Autodesk Fusion 360 part; units mm, degrees
(part 6 of 6)
  arc A719 (142.7278, 4.1602) -> (143.1708, 4.6744) centre (142.6711, 4.657) ccw
  circle A720 centre (0, 0) radius 145
  dimension "d16" = 290
  constraint coincident A720.centre origin
  measures "d16" diameter of A720
extrude "Extrude3" add sketch "Sketch3" along normal blind 2 contours L0 A0 A1 A2 A3 L1 A4 A5 A6 A7 L2 A8 A9 A10 A11 L3 A12 A13 A14 A15 L4 A16 A17 A18 A19 L5 A20 A21 A22 A23 L6 A24 A25 A26 A27 L7 A28 A29 A30 A31 L8 A32 A33 A34 A35 L9 A36 A37 A38 A39 L10 A40 A41 A42 A43 L11 A44 A45 A46 A47 L12 A48 A49 A50 A51 L13 A52 A53 A54 A55 L14 A56 A57 A58 A59 L15 A60 A61 A62 A63 L16 A64 A65 A66 A67 L17 A68 A69 A70 A71 L18 A72 A73 A74 A75 L19 A76 A77 A78 A79 L20 A80 A81 A82 A83 L21 A84 A85 A86 A87 L22 A88 A89 A90 A91 L23 A92 A93 A94 A95 L24 A96 A97 A98 A99 L25 A100 A101 A102 A103 L26 A104 A105 A106 A107 L27 A108 A109 A110 A111 L28 A112 A113 A114 A115 L29 A116 A117 A118 A119 L30 A120 A121 A122 A123 L31 A124 A125 A126 A127 L32 A128 A129 A130 A131 L33 A132 A133 A134 A135 L34 A136 A137 A138 A139 L35 A140 A141 A142 A143 L36 A144 A145 A146 A147 L37 A148 A149 A150 A151 L38 A152 A153 A154 A155 L39 A156 A157 A158 A159 L40 A160 A161 A162 A163 L41 A164 A165 A166 A167 L42 A168 A169 A170 A171 L43 A172 A173 A174 A175 L44 A176 A177 A178 A179 L45 A180 A181 A182 A183 L46 A184 A185 A186 A187 L47 A188 A189 A190 A191 L48 A192 A193 A194 A195 L49 A196 A197 A198 A199 L50 A200 A201 A202 A203 L51 A204 A205 A206 A207 L52 A208 A209 A210 A211 L53 A212 A213 A214 A215 L54 A216 A217 A218 A219 L55 A220 A221 A222 A223 L56 A224 A225 A226 A227 L57 A228 A229 A230 A231 L58 A232 A233 A234 A235 L59 A236 A237 A238 A239 L60 A240 A241 A242 A243 L61 A244 A245 A246 A247 L62 A248 A249 A250 A251 L63 A252 A253 A254 A255 L64 A256 A257 A258 A259 L65 A260 A261 A262 A263 L66 A264 A265 A266 A267 L67 A268 A269 A270 A271 L68 A272 A273 A274 A275 L69 A276 A277 A278 A279 L70 A280 A281 A282 A283 L71 A284 A285 A286 A287 L72 A288 A289 A290 A291 L73 A292 A293 A294 A295 L74 A296 A297 A298 A299 L75 A300 A301 A302 A303 L76 A304 A305 A306 A307 L77 A308 A309 A310 A311 L78 A312 A313 A314 A315 L79 A316 A317 A318 A319 L80 A320 A321 A322 A323 L81 A324 A325 A326 A327 L82 A328 A329 A330 A331 L83 A332 A333 A334 A335 L84 A336 A337 A338 A339 L85 A340 A341 A342 A343 L86 A344 A345 A346 A347 L87 A348 A349 A350 A351 L88 A352 A353 A354 A355 L89 A356 A357 A358 A359 L90 A360 A361 A362 A363 L91 A364 A365 A366 A367 L92 A368 A369 A370 A371 L93 A372 A373 A374 A375 L94 A376 A377 A378 A379 L95 A380 A381 A382 A383 L96 A384 A385 A386 A387 L97 A388 A389 A390 A391 L98 A392 A393 A394 A395 L99 A396 A397 A398 A399 L100 A400 A401 A402 A403 L101 A404 A405 A406 A407 L102 A408 A409 A410 A411 L103 A412 A413 A414 A415 L104 A416 A417 A418 A419 L105 A420 A421 A422 A423 L106 A424 A425 A426 A427 L107 A428 A429 A430 A431 L108 A432 A433 A434 A435 L109 A436 A437 A438 A439 L110 A440 A441 A442 A443 L111 A444 A445 A446 A447 L112 A448 A449 A450 A451 L113 A452 A453 A454 A455 L114 A456 A457 A458 A459 L115 A460 A461 A462 A463 L116 A464 A465 A466 A467 L117 A468 A469 A470 A471 L118 A472 A473 A474 A475 L119 A476 A477 A478 A479 L120 A480 A481 A482 A483 L121 A484 A485 A486 A487 L122 A488 A489 A490 A491 L123 A492 A493 A494 A495 L124 A496 A497 A498 A499 L125 A500 A501 A502 A503 L126 A504 A505 A506 A507 L127 A508 A509 A510 A511 L128 A512 A513 A514 A515 L129 A516 A517 A518 A519 L130 A520 A521 A522 A523 L131 A524 A525 A526 A527 L132 A528 A529 A530 A531 L133 A532 A533 A534 A535 L134 A536 A537 A538 A539 L135 A540 A541 A542 A543 L136 A544 A545 A546 A547 L137 A548 A549 A550 A551 L138 A552 A553 A554 A555 L139 A556 A557 A558 A559 L140 A560 A561 A562 A563 L141 A564 A565 A566 A567 L142 A568 A569 A570 A571 L143 A572 A573 A574 A575 L144 A576 A577 A578 A579 L145 A580 A581 A582 A583 L146 A584 A585 A586 A587 L147 A588 A589 A590 A591 L148 A592 A593 A594 A595 L149 A596 A597 A598 A599 L150 A600 A601 A602 A603 L151 A604 A605 A606 A607 L152 A608 A609 A610 A611 L153 A612 A613 A614 A615 L154 A616 A617 A618 A619 L155 A620 A621 A622 A623 L156 A624 A625 A626 A627 L157 A628 A629 A630 A631 L158 A632 A633 A634 A635 L159 A636 A637 A638 A639 L160 A640 A641 A642 A643 L161 A644 A645 A646 A647 L162 A648 A649 A650 A651 L163 A652 A653 A654 A655 L164 A656 A657 A658 A659 L165 A660 A661 A662 A663 L166 A664 A665 A666 A667 L167 A668 A669 A670 A671 L168 A672 A673 A674 A675 L169 A676 A677 A678 A679 L170 A680 A681 A682 A683 L171 A684 A685 A686 A687 L172 A688 A689 A690 A691 L173 A692 A693 A694 A695 L174 A696 A697 A698 A699 L175 A700 A701 A702 A703 L176 A704 A705 A706 A707 L177 A708 A709 A710 A711 L178 A712 A713 A714 A715 L179 A716 A717 A718 A719 | A720
chamfer "Chamfer1" distance 1.5 angle 45 2 edges at (135.1875, 52.4342, 16) (-135.1875, 52.4342, 0)
sketch "Sketch4" plane through (0, 0, 18) normal (0, 0, 1) x (-1, 0, 0)
  circle A0 centre (0, 0) radius 145
  circle A1 centre (0, 0) radius 110
  dimension "d19" = 220
  constraint coincident A0.centre A1.centre
  measures "d19" diameter of A1
extrude "Extrude4" cut sketch "Sketch4" against normal blind 40 contours A1
sketch "Sketch5" plane through (0, 0, 18) normal (0, 0, 1) x (-1, 0, 0)
  circle A0 centre (0, 0) radius 110
  circle A1 centre (0, 0) radius 145
  line L0 (0, 0) -> (0, -252.5866) construction
  line L1 (0, 0) -> (0, -4.3982) construction
  line L2 (0, 0) -> (-17.5, -126.2933) construction
  line L3 (0, 0) -> (17.5, -126.2933) construction
  circle A2 centre (0, 0) radius 127.5 construction
  line L4 (17.5, -126.2933) -> (-17.5, -126.2933) construction
  line L5 (23.4432, -125.4698) -> (11.5568, -127.1168) construction
  line L6 (25.9047, -128.6621) -> (24.9439, -121.7284)
  line L7 (24.9439, -121.7284) -> (20.9817, -122.2774)
  line L8 (20.9817, -122.2774) -> (21.9425, -129.2112)
  line L9 (21.9425, -129.2112) -> (25.9047, -128.6621)
  line L10 (25.9047, -128.6621) -> (20.9817, -122.2774) construction
  line L11 (13.0575, -123.3755) -> (14.0182, -130.3092)
  line L12 (14.0182, -130.3092) -> (10.0561, -130.8582)
  line L13 (10.0561, -130.8582) -> (9.0953, -123.9245)
  line L14 (9.0953, -123.9245) -> (13.0575, -123.3755)
  line L15 (-21.9425, -129.2112) -> (-25.9047, -128.6621)
  line L16 (-20.9817, -122.2774) -> (-21.9425, -129.2112)
  line L17 (-25.9047, -128.6621) -> (-24.9439, -121.7284)
  line L18 (-24.9439, -121.7284) -> (-20.9817, -122.2774)
  line L19 (-9.0953, -123.9245) -> (-13.0575, -123.3755)
  line L20 (-10.0561, -130.8582) -> (-9.0953, -123.9245)
  line L21 (-13.0575, -123.3755) -> (-14.0182, -130.3092)
  line L22 (-14.0182, -130.3092) -> (-10.0561, -130.8582)
  line L23 (109.2952, -72.6605) -> (103.713, -68.437)
  line L24 (106.8818, -75.8504) -> (109.2952, -72.6605)
  line L25 (101.2995, -71.6269) -> (106.8818, -75.8504)
  line L26 (103.713, -68.437) -> (101.2995, -71.6269)
  line L27 (96.4726, -78.0066) -> (102.0549, -82.2301)
  line L28 (94.0592, -81.1965) -> (96.4726, -78.0066)
  line L29 (99.6415, -85.42) -> (94.0592, -81.1965)
  line L30 (102.0549, -82.2301) -> (99.6415, -85.42)
  line L31 (85.42, -99.6415) -> (81.1965, -94.0592)
  line L32 (82.2301, -102.0549) -> (85.42, -99.6415)
  line L33 (78.0066, -96.4726) -> (82.2301, -102.0549)
  line L34 (81.1965, -94.0592) -> (78.0066, -96.4726)
  line L35 (68.437, -103.713) -> (71.6269, -101.2995)
  line L36 (71.6269, -101.2995) -> (75.8504, -106.8818)
  line L37 (72.6605, -109.2952) -> (68.437, -103.713)
  line L38 (75.8504, -106.8818) -> (72.6605, -109.2952)
  line L39 (128.6621, 25.9047) -> (121.7284, 24.9439)
  line L40 (129.2112, 21.9425) -> (128.6621, 25.9047)
  line L41 (122.2774, 20.9817) -> (129.2112, 21.9425)
  line L42 (121.7284, 24.9439) -> (122.2774, 20.9817)
  line L43 (123.3755, 13.0575) -> (130.3092, 14.0182)
  line L44 (123.9245, 9.0953) -> (123.3755, 13.0575)
  line L45 (130.8582, 10.0561) -> (123.9245, 9.0953)
  line L46 (130.3092, 14.0182) -> (130.8582, 10.0561)
  line L47 (130.8582, -10.0561) -> (123.9245, -9.0953)
  line L48 (130.3092, -14.0182) -> (130.8582, -10.0561)
  line L49 (123.3755, -13.0575) -> (130.3092, -14.0182)
  line L50 (123.9245, -9.0953) -> (123.3755, -13.0575)
  line L51 (121.7284, -24.9439) -> (122.2774, -20.9817)
  line L52 (122.2774, -20.9817) -> (129.2112, -21.9425)
  line L53 (128.6621, -25.9047) -> (121.7284, -24.9439)
  line L54 (129.2112, -21.9425) -> (128.6621, -25.9047)
  line L55 (72.6605, 109.2952) -> (68.437, 103.713)
  line L56 (75.8504, 106.8818) -> (72.6605, 109.2952)
  line L57 (71.6269, 101.2995) -> (75.8504, 106.8818)
  line L58 (68.437, 103.713) -> (71.6269, 101.2995)
  line L59 (78.0066, 96.4726) -> (82.2301, 102.0549)
  line L60 (81.1965, 94.0592) -> (78.0066, 96.4726)
  line L61 (85.42, 99.6415) -> (81.1965, 94.0592)
  line L62 (82.2301, 102.0549) -> (85.42, 99.6415)
  line L63 (99.6415, 85.42) -> (94.0592, 81.1965)
  line L64 (102.0549, 82.2301) -> (99.6415, 85.42)
  line L65 (96.4726, 78.0066) -> (102.0549, 82.2301)
  line L66 (94.0592, 81.1965) -> (96.4726, 78.0066)
  line L67 (103.713, 68.437) -> (101.2995, 71.6269)
  line L68 (101.2995, 71.6269) -> (106.8818, 75.8504)
  line L69 (109.2952, 72.6605) -> (103.713, 68.437)
  line L70 (106.8818, 75.8504) -> (109.2952, 72.6605)
  line L71 (-25.9047, 128.6621) -> (-24.9439, 121.7284)
  line L72 (-21.9425, 129.2112) -> (-25.9047, 128.6621)
  line L73 (-20.9817, 122.2774) -> (-21.9425, 129.2112)
  line L74 (-24.9439, 121.7284) -> (-20.9817, 122.2774)
  line L75 (-13.0575, 123.3755) -> (-14.0182, 130.3092)
  line L76 (-9.0953, 123.9245) -> (-13.0575, 123.3755)
  line L77 (-10.0561, 130.8582) -> (-9.0953, 123.9245)
  line L78 (-14.0182, 130.3092) -> (-10.0561, 130.8582)
  line L79 (10.0561, 130.8582) -> (9.0953, 123.9245)
  line L80 (14.0182, 130.3092) -> (10.0561, 130.8582)
  line L81 (13.0575, 123.3755) -> (14.0182, 130.3092)
  line L82 (9.0953, 123.9245) -> (13.0575, 123.3755)
  line L83 (24.9439, 121.7284) -> (20.9817, 122.2774)
  line L84 (20.9817, 122.2774) -> (21.9425, 129.2112)
  line L85 (25.9047, 128.6621) -> (24.9439, 121.7284)
  line L86 (21.9425, 129.2112) -> (25.9047, 128.6621)
  line L87 (-109.2952, 72.6605) -> (-103.713, 68.437)
  line L88 (-106.8818, 75.8504) -> (-109.2952, 72.6605)
  line L89 (-101.2995, 71.6269) -> (-106.8818, 75.8504)
  line L90 (-103.713, 68.437) -> (-101.2995, 71.6269)
  line L91 (-96.4726, 78.0066) -> (-102.0549, 82.2301)
  line L92 (-94.0592, 81.1965) -> (-96.4726, 78.0066)
  line L93 (-99.6415, 85.42) -> (-94.0592, 81.1965)
  line L94 (-102.0549, 82.2301) -> (-99.6415, 85.42)
  line L95 (-85.42, 99.6415) -> (-81.1965, 94.0592)
  line L96 (-82.2301, 102.0549) -> (-85.42, 99.6415)
  line L97 (-78.0066, 96.4726) -> (-82.2301, 102.0549)
  line L98 (-81.1965, 94.0592) -> (-78.0066, 96.4726)
  line L99 (-68.437, 103.713) -> (-71.6269, 101.2995)
  line L100 (-71.6269, 101.2995) -> (-75.8504, 106.8818)
  line L101 (-72.6605, 109.2952) -> (-68.437, 103.713)
  line L102 (-75.8504, 106.8818) -> (-72.6605, 109.2952)
  line L103 (-128.6621, -25.9047) -> (-121.7284, -24.9439)
  line L104 (-129.2112, -21.9425) -> (-128.6621, -25.9047)
  line L105 (-122.2774, -20.9817) -> (-129.2112, -21.9425)
  line L106 (-121.7284, -24.9439) -> (-122.2774, -20.9817)
  line L107 (-123.3755, -13.0575) -> (-130.3092, -14.0182)
  line L108 (-123.9245, -9.0953) -> (-123.3755, -13.0575)
  line L109 (-130.8582, -10.0561) -> (-123.9245, -9.0953)
  line L110 (-130.3092, -14.0182) -> (-130.8582, -10.0561)
  line L111 (-130.8582, 10.0561) -> (-123.9245, 9.0953)
  line L112 (-130.3092, 14.0182) -> (-130.8582, 10.0561)
  line L113 (-123.3755, 13.0575) -> (-130.3092, 14.0182)
  line L114 (-123.9245, 9.0953) -> (-123.3755, 13.0575)
  line L115 (-121.7284, 24.9439) -> (-122.2774, 20.9817)
  line L116 (-122.2774, 20.9817) -> (-129.2112, 21.9425)
  line L117 (-128.6621, 25.9047) -> (-121.7284, 24.9439)
  line L118 (-129.2112, 21.9425) -> (-128.6621, 25.9047)
  line L119 (-72.6605, -109.2952) -> (-68.437, -103.713)
  line L120 (-75.8504, -106.8818) -> (-72.6605, -109.2952)
  line L121 (-71.6269, -101.2995) -> (-75.8504, -106.8818)
  line L122 (-68.437, -103.713) -> (-71.6269, -101.2995)
  line L123 (-78.0066, -96.4726) -> (-82.2301, -102.0549)
  line L124 (-81.1965, -94.0592) -> (-78.0066, -96.4726)
  line L125 (-85.42, -99.6415) -> (-81.1965, -94.0592)
  line L126 (-82.2301, -102.0549) -> (-85.42, -99.6415)
  line L127 (-99.6415, -85.42) -> (-94.0592, -81.1965)
  line L128 (-102.0549, -82.2301) -> (-99.6415, -85.42)
  line L129 (-96.4726, -78.0066) -> (-102.0549, -82.2301)
  line L130 (-94.0592, -81.1965) -> (-96.4726, -78.0066)
  line L131 (-103.713, -68.437) -> (-101.2995, -71.6269)
  line L132 (-101.2995, -71.6269) -> (-106.8818, -75.8504)
  line L133 (-109.2952, -72.6605) -> (-103.713, -68.437)
  line L134 (-106.8818, -75.8504) -> (-109.2952, -72.6605)
  dimension "d22" = 255
  dimension "d23" = 35
  dimension "d24" = 12
  dimension "d25" = 4
  dimension "d28" = 7
  dimension "d30" = 360
  constraint coincident A0.centre A1.centre
  constraint vertical L0
  constraint coincident L0 L1.end
  constraint concentric A0 A2
  constraint coincident L2.end A2
  constraint coincident L3.end A2
  constraint midpoint L0 L4
  constraint midpoint L3.end L5
  constraint tangent A2 L5
  constraint perpendicular L6 L7
  constraint perpendicular L7 L8
  constraint perpendicular L8 L9
  constraint midpoint L5.start L10
  constraint perpendicular L5 L8
  constraint symmetric L3 L6.start L12.end
  constraint symmetric L3 L6.end L13.end
  constraint symmetric L3 L7.end L11.start
  constraint symmetric L3 L8.end L11.end
  constraint symmetric L0 L6.start L15.end
  constraint symmetric L0 L6.end L17.end
  constraint symmetric L0 L7.end L16.start
  constraint symmetric L0 L8.end L15.start
  constraint symmetric L0 L11.start L19.end
  constraint symmetric L0 L11.end L21.end
  constraint symmetric L0 L12.end L20.start
  constraint symmetric L0 L13.end L19.start
  measures "d22" diameter of A2
  measures "d23" horizontal distance of L2.end L3.end
  measures "d24" distance of L5.start L5.end
  measures "d25" distance of L6.end L7.end
  measures "d28" distance of L7.end L8.end
extrude "Extrude5" cut sketch "Sketch5" against normal through all contours L6 L7 L8 L9 | L11 L12 L13 L14 | L15 L16 L17 L18 | L19 L20 L21 L22 | L23 L24 L25 L26 | L27 L28 L29 L30 | L31 L32 L33 L34 | L35 L36 L37 L38 | L39 L40 L41 L42 | L43 L44 L45 L46 | L47 L48 L49 L50 | L51 L52 L53 L54 | L55 L56 L57 L58 | L59 L60 L61 L62 | L63 L64 L65 L66 | L67 L68 L69 L70 | L71 L72 L73 L74 | L75 L76 L77 L78 | L79 L80 L81 L82 | L83 L84 L85 L86 | L87 L88 L89 L90 | L91 L92 L93 L94 | L95 L96 L97 L98 | L99 L100 L101 L102 | L103 L104 L105 L106 | L107 L108 L109 L110 | L111 L112 L113 L114 | L115 L116 L117 L118 | L119 L120 L121 L122 | L123 L124 L125 L126 | L127 L128 L129 L130 | L131 L132 L133 L134
named bodies: "180Pulley"
